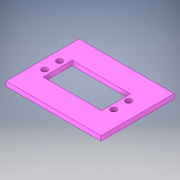
# Autodesk Inventor part: Hombro_servo
Saved by Autodesk Inventor 2019 (Build 230136000, 136)
## iProperties
Created: 2020-02-08
Part Number: Hombro_servo
Material: Generic
Document SubType Name: Modeling
Designer: Omar
Density: 1 g/cm^3
Appearance: Default
Author: Omar
Autodesk Inventor part; units mm, degrees
ref_plane "YZ Plane" through (0, 0, 0) normal (1, 0, 0) x (0, 1, 0)
ref_plane "XZ Plane" through (0, 0, 0) normal (0, 1, 0) x (-1, 0, 0)
ref_plane "XY Plane" through (0, 0, 0) normal (0, 0, 1) x (1, 0, 0)
sketch "Sketch1" plane through (0, 0, 0) normal (0, 1, 0) x (-1, 0, 0)
  circle A0 centre (-33.79, -5.085) radius 2
  circle A1 centre (-33.79, 5.085) radius 2
  circle A2 centre (13.47, -5.085) radius 2
  circle A3 centre (13.47, 5.085) radius 2
  line L0 (20, 25) -> (-45, 25)
  line L1 (-45, 25) -> (-45, -25)
  line L2 (-45, -25) -> (20, -25)
  line L3 (20, -25) -> (20, 25)
  line L4 (9.66, 9.91) -> (-30.22, 9.91)
  line L5 (-30.22, 9.91) -> (-30.22, -9.91)
  line L6 (-30.22, -9.91) -> (9.66, -9.91)
  line L7 (9.66, -9.91) -> (9.66, 9.91)
  point P0 (0, 0)
  point P1 (0, 0)
  dimension "d0" = 4
  dimension "d1" = 4
  dimension "d2" = 4
  dimension "d3" = 4
  dimension "d4" = 13.47
  dimension "d5" = 5.085
  dimension "d6" = 10.17
  dimension "d7" = 13.47
  dimension "d8" = 33.79
  dimension "d9" = 5.085
  dimension "d10" = 10.17
  dimension "d12" = 50
  dimension "d13" = 65
  dimension "d15" = 25
  dimension "d25" = 9.66
  dimension "d26" = 19.82
  dimension "d27" = 9.91
  dimension "d28" = 39.88
  dimension "d29" = 33.79
  dimension "d30" = 20
  constraints: 16 end point, 4 centre point, 4 parallel, 2 horizontal, 2 perpendicular, 1 coincident
  measures "d0" diameter of A0
  measures "d1" diameter of A1
  measures "d2" diameter of A2
  measures "d3" diameter of A3
  measures "d4" horizontal distance of A2.centre point (0, 0)
  measures "d5" vertical distance of A2.centre point (0, 0)
  measures "d6" distance of A3.centre A2.centre
  measures "d7" horizontal distance of point (0, 0) A3.centre
  measures "d8" horizontal distance of A1.centre point (0, 0)
  measures "d9" vertical distance of A1.centre point (0, 0)
  measures "d10" distance of A0.centre A1.centre
  measures "d12" distance of L0.end L1.end
  measures "d13" distance of L0.start L0.end
  measures "d15" distance from line of L0 point (0, 0)
  measures "d25" distance from line of L7 point (0, 0)
  measures "d26" distance of L6.end L4.start
  measures "d27" distance from line of point (0, 0) L6
  measures "d28" distance of L5.end L6.end
  measures "d29" horizontal distance of point (0, 0) A0.centre
  measures "d30" distance from line of L3 point (0, 0)
extrude "Extrusion1" add sketch "Sketch1" along normal blind 3.18
body "Solid1"
